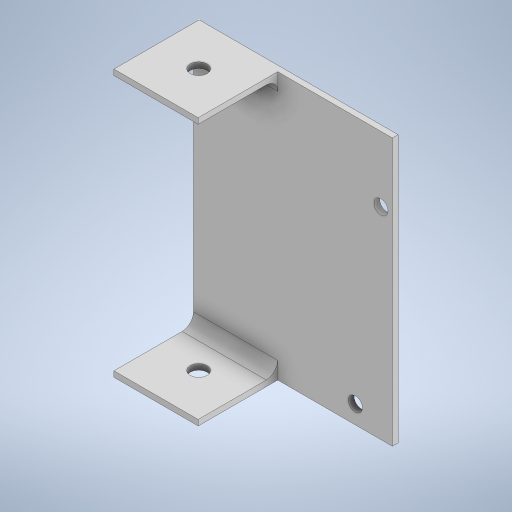
# Autodesk Inventor part: Suportmotor
Saved by Autodesk Inventor 2023 (Build 270158000, 158)
## iProperties
Created: 2022-09-23
Part Number: Suportmotor
Material: Generic
Document SubType Name: Modelado
Designer: hiago.sodre
Density: 1 g/cm^3
Appearance: Default
Sheet Metal Rule: Por defecto_mm
Author: hiago.sodre
Autodesk Inventor part; units mm, degrees
ref_plane "YZ Plane" through (0, 0, 0) normal (1, 0, 0) x (0, 1, 0)
ref_plane "XZ Plane" through (0, 0, 0) normal (0, 1, 0) x (-1, 0, 0)
ref_plane "XY Plane" through (0, 0, 0) normal (0, 0, 1) x (1, 0, 0)
sketch "Sketch12" plane through (0, 0, 0) normal (0, 0, 1) x (1, 0, 0)
  line L0 (0, 0) -> (35, 0)
  line L1 (35, 0) -> (35, 47)
  line L2 (35, 47) -> (0, 47)
  line L3 (0, 47) -> (0, 0)
  line L4 (0, 47) -> (2, 47) construction
  line L5 (2, 47) -> (2, 35.5) construction
  line L6 (35, 47) -> (33, 47) construction
  line L7 (33, 47) -> (33, 35.5) construction
  circle A0 centre (33, 35.5) radius 1.25
  circle A1 centre (2, 35.5) radius 1.25
  line L8 (0, 0) -> (6.5, 0) construction
  line L9 (35, 0) -> (28.5, 0) construction
  line L10 (6.5, 0) -> (6.5, 3.2) construction
  line L11 (28.5, 0) -> (28.5, 3.2) construction
  circle A2 centre (28.5, 3.2) radius 1.25
  dimension "d49" = 35
  dimension "d50" = 47
  dimension "d97" = 2
  dimension "d98" = 11.5
  dimension "d99" = 2
  dimension "d100" = 2.5
  dimension "d101" = 2.5
  dimension "d102" = 11.5
  dimension "d103" = 6.5
  dimension "d104" = 6.5
  dimension "d105" = 3.2
  dimension "d106" = 3.2
  dimension "d108" = 2.5
  constraints: 24 end point, 4 point on line, 3 centre point, 3 coincident, 3 perpendicular, 2 parallel, 2 vertical, 1 horizontal
  measures "d49" distance of L2.end L1.end
  measures "d50" distance of L1.end L0.end
  measures "d97" distance of L2.end L4.end
  measures "d98" distance of L4.end L5.end
  measures "d99" distance of L1.end L6.end
  measures "d100" diameter of A0
  measures "d101" diameter of A1
  measures "d102" distance of L6.end L7.end
  measures "d103" distance of L0.start L8.end
  measures "d104" distance of L0.end L9.end
  measures "d105" distance of L8.end L10.end
  measures "d106" distance of L9.end L11.end
  measures "d108" diameter of A2
extrude "Extrusión8" add sketch "Sketch12" along normal blind 1
sketch "Sketch25" plane through (0, 47, 0) normal (0, 1, 0) x (1, 0, 0)
  point P0 (0, 0)
sketch "Sketch26" plane through (0, 0, 0) normal (0, -1, 0) x (1, 0, 0)
  line L0 (35, 1) -> (20.1754, 1)
  line L1 (20.1754, 1) -> (20.1754, 15)
  line L2 (20.1754, 15) -> (35, 15)
  line L3 (35, 15) -> (35, 1)
  line L4 (0, 1) -> (14.825, 1)
  line L5 (35, 1) -> (0, 1) projected
  line L6 (14.825, 1) -> (14.825, 15)
  line L7 (14.825, 15) -> (0, 15)
  line L8 (0, 15) -> (0, 1)
  point P0 (0, 0)
  dimension "d121" = 14.825
  dimension "d126" = 14
  constraints: 16 end point, 4 perpendicular, 2 parallel, 2 point on line, 1 horizontal
  measures "d121" distance of L4.start L4.end
  measures "d126" distance of L4.end L6.end
extrude "Extrusion10" add sketch "Sketch26" against normal blind 1 contours L4 L8 L7 L6
fillet "Empalme1" radius 2 1 edges at (7.4125, 1, 1)
sketch "Boceto28" plane through (0, 47, 0) normal (0, 1, 0) x (1, 0, 0)
  line L0 (0, 0) -> (0, -1) projected
  line L1 (0, -1) -> (14.825, -1)
  line L2 (0, -3) -> (14.825, -3) projected
  line L3 (14.825, -15) -> (14.825, -3) projected
  line L4 (14.825, -1) -> (14.825, -15)
  line L5 (0, -15) -> (14.825, -15) projected
  line L6 (14.825, -15) -> (0, -15)
  line L7 (0, -15) -> (0, -1)
  point P0 (14.825, -3)
  constraints: 8 end point, 2 equal length, 2 perpendicular
extrude "Extrusión12" add sketch "Boceto28" against normal blind 1
fillet "Empalme2" radius 2 1 edges at (7.4125, 46, 1)
sketch "Boceto29" plane through (0, 47, 0) normal (0, 1, 0) x (1, 0, 0)
  line L0 (0, 0) -> (0, -15) projected
  line L1 (0, -7.5) -> (14.825, -7.5)
  line L2 (14.825, -15) -> (14.825, -3) projected
  line L3 (7.4125, -7.5) -> (7.4125, -15)
  line L4 (0, -15) -> (14.825, -15) projected
  circle A0 centre (7.4125, -7.5) radius 1.5
  dimension "d127" = 3
  constraints: 4 end point, 3 midpoint, 1 centre point, 1 coincident, 1 horizontal, 1 point on line
  measures "d127" diameter of A0
extrude "Extrusión13" cut sketch "Boceto29" against normal through all contours A0 L1 | L1 L3 A0 | L1 A0 L3
equation "\"BendRadius\" = Thickness"
equation "\"BendReliefWidth\" = Thickness"
equation "\"BendReliefDepth\" = 0.5 * Thickness"
equation "\"CornerReliefSize\" = 4 * Thickness"
equation "\"MinimumRemnant\" = 2 * Thickness"
equation "\"TransitionRadius\" = BendRadius"
equation "\"JacobiRadiusSize\" = BendRadius"
equation "\"GapSize\" = Thickness"
equation "\"Thickness\" = 1"
